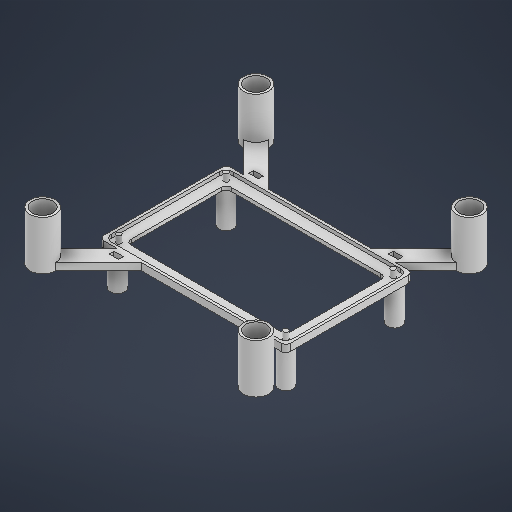
# Autodesk Inventor part: Drone
Saved by Autodesk Inventor 2026 (Build 300175050, 175E)
## iProperties
Created: 2026-01-22
Part Number: Drone
Material: Ogólny
Document SubType Name: Modeling
Designer: DeathLock
Density: 1 g/cm^3
Appearance: Domyślna
Author: DeathLock
Autodesk Inventor part; units mm, degrees
ref_plane "YZ Plane" through (0, 0, 0) normal (1, 0, 0) x (0, 1, 0)
ref_plane "XZ Plane" through (0, 0, 0) normal (0, 1, 0) x (-1, 0, 0)
ref_plane "XY Plane" through (0, 0, 0) normal (0, 0, 1) x (1, 0, 0)
sketch "Szkic1" plane through (0, 0, 0) normal (0, 1, 0) x (-1, 0, 0)
  line L0 (50, 50) -> (-50, 50)
  line L1 (-50, 50) -> (-50, -50)
  line L2 (-50, -50) -> (50, -50)
  line L3 (50, -50) -> (50, 50)
  point P0 (0, 0)
  dimension "d71" = 50
  dimension "d72" = 50
  dimension "d73" = 50
  dimension "d74" = 50
  constraints: 8 end point, 2 parallel, 1 horizontal, 1 perpendicular
  measures "d71" distance from line of L2 point (0, 0)
  measures "d72" distance from line of L3 point (0, 0)
  measures "d73" distance from line of L0 point (0, 0)
  measures "d74" distance from line of L1 point (0, 0)
extrude "Wyciągnięcie proste1" add sketch "Szkic1" along normal blind 3
sketch "Szkic2" plane through (0, 3, 0) normal (0, 1, 0) x (1, 0, 0)
  line L0 (-50, 50) -> (-50, -50) projected
  line L1 (-50, 0) -> (50, 0)
  line L2 (50, -50) -> (50, 50) projected
  line L3 (-38, -25.5) -> (38, -25.5)
  line L4 (38, -25.5) -> (38, 25.5)
  line L5 (38, 25.5) -> (-38, 25.5)
  line L6 (-38, 25.5) -> (-38, -25.5)
  line L7 (-50, -50) -> (50, -50) projected
  line L8 (50, 50) -> (-50, 50) projected
  line L9 (-38, -25.5) -> (-35, -25.5)
  line L10 (-35, -25.5) -> (-35, -22.5)
  line L11 (-35, -22.5) -> (-38, -22.5)
  line L12 (-38, -22.5) -> (-38, -25.5)
  line L13 (-38, 25.5) -> (-35, 25.5)
  line L14 (-35, 25.5) -> (-35, 22.5)
  line L15 (-35, 22.5) -> (-38, 22.5)
  line L16 (-38, 22.5) -> (-38, 25.5)
  line L17 (38, -25.5) -> (35, -25.5)
  line L18 (35, -25.5) -> (35, -22.5)
  line L19 (35, -22.5) -> (38, -22.5)
  line L20 (38, -22.5) -> (38, -25.5)
  line L21 (38, 25.5) -> (35, 25.5)
  line L22 (35, 25.5) -> (35, 22.5)
  line L23 (35, 22.5) -> (38, 22.5)
  line L24 (38, 22.5) -> (38, 25.5)
  circle A0 centre (-35, -22.5) radius 3
  circle A1 centre (-35, 22.5) radius 3
  circle A2 centre (35, 22.5) radius 3
  circle A3 centre (35, -22.5) radius 3
  point P0 (0, 0)
  point P1 (0, -25.5)
  point P2 (0, 25.5)
  point P3 (-38, 0)
  point P4 (38, 0)
  point P5 (-35, -25.5)
  point P6 (38, 22.5)
  dimension "d4" = 76
  dimension "d5" = 51
  dimension "d6" = 24.5
  dimension "d7" = 24.5
  dimension "d8" = 12
  dimension "d9" = 12
  dimension "d10" = 3
  dimension "d11" = 3
  dimension "d12" = 3
  dimension "d13" = 3
  dimension "d14" = 3
  dimension "d15" = 3
  dimension "d16" = 3
  dimension "d17" = 3
  dimension "d75" = 12
  constraints: 42 end point, 10 parallel, 6 midpoint, 5 horizontal, 5 perpendicular, 4 coincident, 12 other
  measures "d4" distance of L5.end L4.end
  measures "d5" distance of L4.end L3.end
  measures "d6" distance from line of L7 point (0, -25.5)
  measures "d7" distance from line of L8 point (0, 25.5)
  measures "d8" distance from line of L0 point (-38, 0)
  measures "d9" distance from line of L2 point (38, 0)
  measures "d10" distance of L11.end L10.end
  measures "d11" distance of L10.end L9.end
  measures "d12" distance of L14.end L15.end
  measures "d13" distance of L13.end L14.end
  measures "d14" distance of L18.end L19.end
  measures "d15" distance of L17.end L18.end
  measures "d16" distance of L23.end L22.end
  measures "d17" distance of L22.end L21.end
  measures "d75" distance between parallel lines of L2 L4
extrude "Wyciągnięcie proste2" cut sketch "Szkic2" against normal blind 1.5 contours L6 A1 L5 A2 L4 L1 | L1 L4 A3 L3 A0 L6 | A1 L14 L15 | L15 L14 A1 | A0 L10 L11 | L11 L10 A0 | A3 L18 L19 | L19 L18 A3 | A2 L22 L23 | L23 L22 A2
sketch "Szkic3" plane through (0, 1.5, 0) normal (0, 1, 0) x (1, 0, 0)
  arc A0 (-38, -22.5) -> (-35, -25.5) centre (-35, -22.5) ccw projected
  arc A1 (38, 22.5) -> (35, 25.5) centre (35, 22.5) ccw projected
  line L0 (-35, -25.5) -> (35, -25.5)
  line L1 (35, -25.5) -> (35, 25.5)
  line L2 (35, 25.5) -> (-35, 25.5)
  line L3 (-35, 25.5) -> (-35, -25.5)
  line L4 (-38, -22.5) -> (-38, 22.5) projected
  line L5 (38, 22.5) -> (-38, 22.5)
  line L6 (-38, 22.5) -> (-38, -22.5)
  line L7 (-38, -22.5) -> (38, -22.5)
  line L8 (38, -22.5) -> (38, 22.5)
  circle A2 centre (-35, -22.5) radius 1
  circle A3 centre (-35, 22.5) radius 1
  circle A4 centre (35, -22.5) radius 1
  circle A5 centre (35, 22.5) radius 1
  point P0 (0, 0)
  dimension "d20" = 2
  dimension "d21" = 2
  dimension "d22" = 2
  dimension "d23" = 2
  constraints: 16 end point, 4 centre point, 4 parallel, 4 point on line, 2 coincident, 2 horizontal, 2 perpendicular
  measures "d20" diameter of A2
  measures "d21" diameter of A3
  measures "d22" diameter of A4
  measures "d23" diameter of A5
extrude "Wyciągnięcie proste3" add sketch "Szkic3" along normal blind 3 contours A2 L3 L7 | L7 L3 A2 | L3 L7 A2 | A3 L3 L5 | L5 L3 A3 | L3 A2 L7 | A4 L7 L1 | L1 L7 A4 | L5 A3 L3 | L3 A3 L5 | L7 A4 L1 | L1 A4 L7 | A5 L1 L5 | L5 L1 A5 | L1 L5 A5 | L1 A5 L5
sketch "Szkic7" plane through (0, 1.5, 0) normal (0, 1, 0) x (1, 0, 0)
  arc A0 (-38, -22.5) -> (-35, -25.5) centre (-35, -22.5) ccw projected
  line L0 (38, 22.5) -> (38, -22.5) projected
  line L1 (-38, -22.5) -> (38, -22.5)
  line L2 (38, -22.5) -> (38, 22.5)
  line L3 (38, 22.5) -> (-38, 22.5)
  line L4 (-38, 22.5) -> (-38, -22.5)
  arc A1 (38, 22.5) -> (35, 25.5) centre (35, 22.5) ccw projected
  line L5 (35, 25.5) -> (-35, 25.5)
  line L6 (-35, 25.5) -> (-35, -25.5)
  line L7 (-35, -25.5) -> (35, -25.5)
  line L8 (35, -25.5) -> (35, 25.5)
  line L9 (-35, -22.5) -> (-32.8787, -20.3787)
  line L10 (-35, -22.5) -> (-32, -22.5) construction
  line L11 (35, 22.5) -> (32.8787, 20.3787)
  line L12 (35, -22.5) -> (32.8787, -20.3787)
  circle A2 centre (-35, 22.5) radius 1 projected
  line L13 (-35, 22.5) -> (-32.8787, 20.3787)
  line L14 (-32.8787, -20.3787) -> (32.8787, -20.3787)
  line L15 (32.8787, -20.3787) -> (32.8787, 20.3787)
  line L16 (32.8787, 20.3787) -> (-32.8787, 20.3787)
  line L17 (-32.8787, 20.3787) -> (-32.8787, -20.3787)
  line L18 (-32.8787, -20.3787) -> (-31.3789, -18.8789)
  circle A3 centre (-31.3789, -18.8789) radius 2.121
  line L19 (-32.8787, 20.3787) -> (-31.3789, 18.8789)
  line L20 (32.8787, 20.3787) -> (31.3789, 18.8789)
  line L21 (32.8787, -20.3787) -> (31.3789, -18.8789)
  circle A4 centre (-31.3789, 18.8789) radius 2.121
  circle A5 centre (31.3789, 18.8789) radius 2.121
  circle A6 centre (31.3789, -18.8789) radius 2.121
  line L22 (31.3789, -20.9999) -> (-31.3789, -20.9999)
  line L23 (-31.3789, -20.9999) -> (-31.3789, 20.9999)
  line L24 (-31.3789, 20.9999) -> (31.3789, 20.9999)
  line L25 (31.3789, 20.9999) -> (31.3789, -20.9999)
  line L26 (-33.4999, 18.8789) -> (33.4999, 18.8789)
  line L27 (33.4999, 18.8789) -> (33.4999, -18.8789)
  line L28 (33.4999, -18.8789) -> (-33.4999, -18.8789)
  line L29 (-33.4999, -18.8789) -> (-33.4999, 18.8789)
  point P0 (0, 0)
  point P1 (-33.4999, -18.8789)
  point P2 (-31.3789, -20.9999)
  point P3 (33.4999, 18.8789)
  point P4 (31.3789, 20.9999)
  dimension "d56" = 3
  dimension "d57" = 45
  dimension "d58" = 3
  dimension "d59" = 3
  dimension "d60" = 3
  dimension "d61" = 2.121
  dimension "d62" = 2.121
  dimension "d63" = 2.121
  dimension "d64" = 2.121
  constraints: 58 end point, 10 parallel, 6 horizontal, 6 point on circle, 5 perpendicular, 4 coincident, 2 centre point, 2 point on line, 1 equal length, 6 other
  measures "d56" distance of L9.start L9.end
  measures "d57" angle of L10 L9
  measures "d58" distance of L11.start L11.end
  measures "d59" distance of L12.start L12.end
  measures "d60" distance of L13.start L13.end
  measures "d61" distance of L9.end L18.end
  measures "d62" distance of L16.end L19.end
  measures "d63" distance of L11.end L20.end
  measures "d64" distance of L14.end L21.end
extrude "Wyciągnięcie proste6" cut sketch "Szkic7" against normal blind 17.5 contours L18 L23 L14 | A3 L28 L17 | L17 L28 L18 | L14 L23 A3 | A6 L25 L14 | L21 L28 L15 | L14 L25 L21 | L15 L28 A6 | L23 L28 A3 L14 | L14 A3 L23 | L28 A3 L17 | L17 A3 L23 L28 | L23 A3 L28 | L29 A4 L17 A3 | A3 L14 A6 L22 | A5 L26 L15 | L20 L25 L16 | L15 L26 L20 | L16 L25 A5 | L25 A6 L14 | L14 A6 L28 L25 | L28 L25 A6 L15 | L15 A6 L28 | L28 A6 L25 | A6 L15 A5 L27 | A4 L23 L16 | L19 L26 L17 | L16 L23 L19 | L17 L26 A4 | A3 L28 A6 L14 | L17 A4 L23 A3 | L23 A4 L26 A5 L25 A6 L28 A3 | L26 L17 A4 | L26 A5 L15 | L15 A5 L25 L26 | L25 L26 A5 L16 | L16 A5 L25 | L25 A5 L26 | A5 L16 A4 L24 | A6 L25 A5 L15 | L23 A4 L16 | L16 A4 L26 L23 | L26 L23 A4 L17 | L26 A4 L23 | A5 L26 A4 L16
sketch "Szkic10" plane through (0, 3, 0) normal (0, 1, 0) x (1, 0, 0)
  line L0 (50, 50) -> (-50, 50) projected
  line L1 (-35, 25.5) -> (35, 25.5) projected
  line L2 (-50, -50) -> (50, -50) projected
  line L3 (35, -25.5) -> (-35, -25.5) projected
  line L4 (50, -50) -> (50, 50) projected
  line L5 (38, 22.5) -> (38, -22.5) projected
  line L6 (-38, -22.5) -> (-38, 22.5) projected
  line L7 (-50, 50) -> (-50, -50) projected
  line L8 (50, 50) -> (44.7, 50)
  line L9 (44.7, 50) -> (44.7, 44.7)
  line L10 (44.7, 44.7) -> (50, 44.7)
  line L11 (50, 44.7) -> (50, 50)
  line L12 (-50, 50) -> (-44.7, 50)
  line L13 (-44.7, 50) -> (-44.7, 44.7)
  line L14 (-44.7, 44.7) -> (-50, 44.7)
  line L15 (-50, 44.7) -> (-50, 50)
  line L16 (-50, -50) -> (-44.7, -50)
  line L17 (-44.7, -50) -> (-44.7, -44.7)
  line L18 (-44.7, -44.7) -> (-50, -44.7)
  line L19 (-50, -44.7) -> (-50, -50)
  line L20 (50, -50) -> (44.7, -50)
  line L21 (44.7, -50) -> (44.7, -44.7)
  line L22 (44.7, -44.7) -> (50, -44.7)
  line L23 (50, -44.7) -> (50, -50)
  circle A0 centre (-44.7, -44.7) radius 5.3
  circle A1 centre (44.7, -44.7) radius 5.3
  circle A2 centre (44.7, 44.7) radius 5.3
  circle A3 centre (-44.7, 44.7) radius 5.3
  circle A4 centre (-44.7, 44.7) radius 4.3
  circle A5 centre (44.7, 44.7) radius 4.3
  circle A6 centre (44.7, -44.7) radius 4.3
  circle A7 centre (-44.7, -44.7) radius 4.3
  point P0 (0, 0)
  dimension "d76" = 24.5
  dimension "d77" = 24.5
  dimension "d78" = 12
  dimension "d79" = 12
  dimension "d80" = 5.3
  dimension "d81" = 5.3
  dimension "d82" = 5.3
  dimension "d83" = 5.3
  dimension "d84" = 5.3
  dimension "d85" = 5.3
  dimension "d86" = 5.3
  dimension "d87" = 5.3
  dimension "d88" = 10.6
  dimension "d89" = 10.6
  dimension "d90" = 10.6
  dimension "d91" = 10.6
  dimension "d92" = 8.6
  dimension "d93" = 8.6
  dimension "d94" = 8.6
  dimension "d95" = 8.6
  constraints: 32 end point, 8 centre point, 8 coincident, 8 parallel, 4 horizontal, 4 perpendicular
  measures "d76" distance between parallel lines of L0 L1
  measures "d77" distance between parallel lines of L2 L3
  measures "d78" distance between parallel lines of L4 L5
  measures "d79" distance between parallel lines of L6 L7
  measures "d80" distance of L10.end L9.end
  measures "d81" distance of L9.end L8.end
  measures "d82" distance of L13.end L14.end
  measures "d83" distance of L12.end L13.end
  measures "d84" distance of L18.end L17.end
  measures "d85" distance of L17.end L16.end
  measures "d86" distance of L21.end L22.end
  measures "d87" distance of L20.end L21.end
  measures "d88" diameter of A0
  measures "d89" diameter of A1
  measures "d90" diameter of A2
  measures "d91" diameter of A3
  measures "d92" diameter of A4
  measures "d93" diameter of A5
  measures "d94" diameter of A6
  measures "d95" diameter of A7
extrude "Wyciągnięcie proste8" add sketch "Szkic10" along normal blind 17.5 contours A2 L10 A5 L9 | L9 A5 L10 A2 | A3 L14 A4 L13 | L13 A4 L14 A3 | A1 L21 A6 L22 | L22 A6 L21 A1 | A0 L17 A7 L18 | L18 A7 L17 A0
sketch "Szkic11" plane through (0, 3, 0) normal (0, 1, 0) x (1, 0, 0)
  arc A0 (-44.7, -50) -> (-50, -44.7) centre (-44.7, -44.7) ccw projected
  arc A1 (-50, -44.7) -> (-44.7, -50) centre (-44.7, -44.7) ccw projected
  line L0 (-40.6047, -41.3357) -> (-44.7, -44.7)
  circle A2 centre (44.7, -44.7) radius 5.3 projected
  line L1 (41.3934, -40.558) -> (44.7, -44.7)
  circle A3 centre (44.7, 44.7) radius 4.3 projected
  line L2 (44.7, 40.4) -> (44.7, 44.7)
  circle A4 centre (-44.7, 44.7) radius 4.3 projected
  line L3 (-48.3948, 42.5003) -> (-44.7, 44.7)
  circle A5 centre (-44.7, 44.7) radius 5.3 projected
  line L4 (-50, 50) -> (-50, 44.7) projected
  arc A6 (-44.7, 50) -> (-50, 44.7) centre (-44.7, 44.7) ccw
  line L5 (50, -50) -> (50, 50) projected
  line L6 (50, 50) -> (44.7, 50) projected
  arc A7 (50, 44.7) -> (44.7, 50) centre (44.7, 44.7) ccw
  arc A8 (44.7, -50) -> (50, -44.7) centre (44.7, -44.7) ccw
  arc A9 (-50, -44.7) -> (-44.7, -50) centre (-44.7, -44.7) ccw
  line L7 (-50, -44.7) -> (-50, -50) projected
  line L8 (-50, -50) -> (-44.7, -50)
  line L9 (-44.7, -50) -> (-44.7, -44.7)
  line L10 (-44.7, -44.7) -> (-50, -44.7)
  line L11 (-50, -44.7) -> (-50, -50)
  line L12 (44.7, -44.7) -> (50, -44.7)
  line L13 (50, -44.7) -> (50, -50)
  line L14 (50, -50) -> (44.7, -50)
  line L15 (44.7, -50) -> (44.7, -44.7)
  line L16 (44.7, 44.7) -> (50, 44.7)
  line L17 (50, 44.7) -> (50, 50)
  line L18 (50, 50) -> (44.7, 50)
  line L19 (44.7, 50) -> (44.7, 44.7)
  line L20 (-50, 50) -> (-44.7, 50)
  line L21 (-44.7, 50) -> (-44.7, 44.7)
  line L22 (-44.7, 44.7) -> (-50, 44.7)
  line L23 (-50, 44.7) -> (-50, 50)
  point P0 (0, 0)
  constraints: 40 end point, 13 point on circle, 8 parallel, 4 centre point, 4 coincident, 4 horizontal, 4 perpendicular, 2 point on line, 1 concentric, 1 vertical, 1 vertical alignment, 3 other
extrude "Wyciągnięcie proste9" cut sketch "Szkic11" against normal blind 17.5 contours L8 L7 A1 | L5 L14 A2 | A7 L6 L5 | L4 L20 A5
sketch "Szkic12" plane through (0, 3, 0) normal (0, 1, 0) x (1, 0, 0)
  circle A0 centre (-44.7, 44.7) radius 4.3 projected
  line L0 (-49, 44.7) -> (-40.4, 44.7)
  arc A1 (44.7, 50) -> (50, 44.7) centre (44.7, 44.7) ccw projected
  line L1 (44.7, 44.7) -> (40.4, 44.7)
  circle A2 centre (44.7, 44.7) radius 4.3 projected
  line L2 (44.7, 44.7) -> (49, 44.7)
  circle A3 centre (44.7, -44.7) radius 4.3 projected
  line L3 (44.7, -44.7) -> (40.4, -44.7)
  line L4 (44.7, -44.7) -> (49, -44.7)
  line L5 (-44.7, -44.7) -> (-40.4, -44.7)
  line L6 (-40.4, -44.7) -> (-44.7, -44.7)
  circle A4 centre (-44.7, -44.7) radius 4.3 projected
  line L7 (-44.7, -44.7) -> (-49, -44.7)
  arc A5 (-50, -44.7) -> (-44.7, -50) centre (-44.7, -44.7) ccw projected
  line L8 (-50, -44.7) -> (-39.4952, -44.7)
  line L9 (-39.4952, -44.7) -> (-39.4952, -43.7)
  line L10 (-39.4952, -43.7) -> (-50, -43.7)
  line L11 (-50, -43.7) -> (-50, -44.7)
  line L12 (-50, -44.7) -> (-39.4952, -44.7)
  line L13 (-39.4952, -44.7) -> (-39.4952, -45.7)
  line L14 (-39.4952, -45.7) -> (-50, -45.7)
  line L15 (-50, -45.7) -> (-50, -44.7)
  arc A6 (50, -44.7) -> (44.7, -50) centre (44.7, -44.7) ccw projected
  line L16 (49, -44.7) -> (39.4952, -44.7)
  line L17 (39.4952, -44.7) -> (39.4952, -43.7)
  line L18 (39.4952, -43.7) -> (49, -43.7)
  line L19 (49, -43.7) -> (49, -44.7)
  line L20 (49, -44.7) -> (39.4952, -44.7)
  line L21 (39.4952, -44.7) -> (39.4952, -45.7)
  line L22 (39.4952, -45.7) -> (49, -45.7)
  line L23 (49, -45.7) -> (49, -44.7)
  line L24 (40.4, 44.7) -> (49.9048, 44.7)
  line L25 (49.9048, 44.7) -> (49.9048, 45.7)
  line L26 (49.9048, 45.7) -> (40.4, 45.7)
  line L27 (40.4, 45.7) -> (40.4, 44.7)
  line L28 (50, -44.7) -> (50, 44.7) projected
  line L29 (40.4, 44.7) -> (50, 44.7)
  line L30 (50, 44.7) -> (50, 43.7)
  line L31 (50, 43.7) -> (40.4, 43.7)
  line L32 (40.4, 43.7) -> (40.4, 44.7)
  line L33 (-49, 44.7) -> (-39.4952, 44.7)
  line L34 (-39.4952, 44.7) -> (-39.4952, 45.7)
  line L35 (-39.4952, 45.7) -> (-49, 45.7)
  line L36 (-49, 45.7) -> (-49, 44.7)
  line L37 (-49, 44.7) -> (-39.4952, 44.7)
  line L38 (-39.4952, 44.7) -> (-39.4952, 43.7)
  line L39 (-39.4952, 43.7) -> (-49, 43.7)
  line L40 (-49, 43.7) -> (-49, 44.7)
  point P0 (0, 0)
  point P1 (-40.5179, -43.7)
  point P2 (-48.8821, -43.7)
  point P3 (-48.8821, -45.7)
  point P4 (-40.5179, -45.7)
  point P5 (48.8821, -43.7)
  point P6 (40.5179, -43.7)
  point P7 (40.5179, -45.7)
  point P8 (48.8821, -45.7)
  point P9 (48.8821, 45.7)
  point P10 (40.5179, 45.7)
  point P11 (40.5179, 43.7)
  point P12 (48.8821, 43.7)
  point P13 (-48.8821, 43.7)
  point P14 (-40.5179, 43.7)
  point P15 (-40.5179, 45.7)
  point P16 (-48.8821, 45.7)
  dimension "d100" = 1
  dimension "d101" = 1
  dimension "d102" = 1
  dimension "d103" = 1
  dimension "d104" = 1
  dimension "d105" = 1
  dimension "d106" = 1
  dimension "d107" = 1
  constraints: 80 end point, 18 equal length, 12 point on circle, 9 horizontal, 9 point on line, 8 perpendicular
  measures "d100" distance of L9.end L8.end
  measures "d101" distance of L12.end L13.end
  measures "d102" distance of L16.end L17.end
  measures "d103" distance of L21.end L20.end
  measures "d104" distance of L25.end L24.end
  measures "d105" distance of L29.end L30.end
  measures "d106" distance of L34.end L33.end
  measures "d107" distance of L37.end L38.end
extrude "Wyciągnięcie proste10" cut sketch "Szkic12" against normal blind 17.5 contours L0 A0 L35 | A0 L39 L0 | L31 A2 L1 L2 | L2 L1 A2 L26 | L4 L3 A3 L18 | A3 L22 L3 L4 | L7 A4 L10 L5 | L5 A4 L14 L7
sketch "Szkic14" plane through (0, 3, 0) normal (0, 1, 0) x (1, 0, 0)
  circle A0 centre (-35, 22.5) radius 1 projected
  line L0 (-35, 22.5) -> (-37.1213, 24.6213)
  arc A1 (-35, 25.5) -> (-38, 22.5) centre (-35, 22.5) ccw projected
  line L1 (-35, 22.5) -> (-32, 22.5) construction
  line L2 (-37.1213, 24.6213) -> (-38.5355, 26.0355)
  line L3 (-37.1213, 24.6213) -> (-35.1213, 24.6213) construction
  circle A2 centre (-37.1213, 24.6213) radius 2
  arc A3 (38, 22.5) -> (35, 25.5) centre (35, 22.5) ccw projected
  circle A4 centre (37.1213, 24.6213) radius 2
  arc A5 (35, -25.5) -> (38, -22.5) centre (35, -22.5) ccw projected
  circle A6 centre (37.1213, -24.6213) radius 2
  arc A7 (-38, -22.5) -> (-35, -25.5) centre (-35, -22.5) ccw projected
  circle A8 centre (-37.1213, -24.6213) radius 2
  line L4 (-39.1213, -24.6213) -> (-39.1213, 24.6213)
  line L5 (-37.1213, 26.6213) -> (37.1213, 26.6213)
  line L6 (39.1213, 24.6213) -> (39.1213, -24.6213)
  line L7 (37.1213, -26.6213) -> (-37.1213, -26.6213)
  line L8 (-50, 44.7) -> (-50, -44.7) projected
  line L9 (50, -44.7) -> (50, 44.7) projected
  line L10 (-50, 44.7) -> (50, 44.7)
  line L11 (50, 44.7) -> (50, -44.7)
  line L12 (50, -44.7) -> (-50, -44.7)
  line L13 (-50, -44.7) -> (-50, 44.7)
  circle A9 centre (44.7, -44.7) radius 5.3 projected
  circle A10 centre (-44.7, 44.7) radius 5.3 projected
  line L14 (44.7, -50) -> (-44.7, -50)
  line L15 (-44.7, -50) -> (-44.7, 50)
  line L16 (-44.7, 50) -> (44.7, 50)
  line L17 (44.7, 50) -> (44.7, -50)
  circle A11 centre (-44.7, -44.7) radius 5.3
  circle A12 centre (44.7, -44.7) radius 5.3
  circle A13 centre (44.7, 44.7) radius 5.3
  circle A14 centre (-44.7, 44.7) radius 5.3
  line L18 (-32, -26.6213) -> (-21.3769, -26.6213)
  line L19 (-44.7, -39.4) -> (-34, -39.4)
  arc A15 (-48.8821, -43.7) -> (-48.8821, -45.7) centre (-44.7, -44.7) ccw projected
  line L20 (-48.8821, -43.7) -> (-43.7, -48.8821)
  arc A16 (-48.8821, -45.7) -> (-40.5179, -45.7) centre (-44.7, -44.7) ccw projected
  circle A17 centre (-44.7, 44.7) radius 4.3 projected
  line L21 (-48.8821, 43.7) -> (-43.7, 48.8821)
  circle A18 centre (44.7, 44.7) radius 4.3 projected
  line L22 (43.7, 48.8821) -> (48.8821, 43.7)
  circle A19 centre (44.7, -44.7) radius 4.3 projected
  line L23 (43.7, -48.8821) -> (48.8821, -43.7)
  line L24 (-44.7, 39.4) -> (39.4, -44.7)
  line L25 (44.7, -39.4) -> (-39.4, 44.7)
  line L26 (39.4, 44.7) -> (-44.7, -39.4)
  line L27 (-39.4, -44.7) -> (44.7, 39.4)
  point P0 (0, 0)
  point P1 (31.9213, -26.6213)
  point P2 (31.9213, 26.6213)
  point P3 (21.3213, 26.6213)
  point P4 (-39.4, 44.7)
  point P5 (-21.3213, 26.6213)
  point P6 (21.3213, -26.6213)
  point P7 (-21.3213, -26.6213)
  point P8 (-31.9213, -26.6213)
  point P9 (-31.9213, 26.6213)
  point P10 (-44.7, 39.4)
  point P11 (-50, -44.7)
  dimension "d118" = 135
  dimension "d119" = 2
  dimension "d120" = 135
  dimension "d121" = 4
  dimension "d122" = 4
  dimension "d123" = 4
  constraints: 52 end point, 30 point on circle, 13 point on line, 8 centre point, 6 parallel, 6 tangent, 5 perpendicular, 4 horizontal, 3 coincident, 2 concentric, 2 equal length, 1 collinear
  measures "d118" angle of L1 L0
  measures "d119" distance of L0.end L2.end
  measures "d120" angle of L3 L2
  measures "d121" diameter of A4
  measures "d122" diameter of A6
  measures "d123" diameter of A8
extrude "Wyciągnięcie proste11" cut sketch "Szkic14" against normal blind 17.5 contours A2 L4 A8 L7 L26 L15 L24 L5 | L25 L10 L26 L5 | L15 A11 L8 A10 | A10 L16 A13 L10 | L27 L17 L25 L7 A6 L6 A4 L5 | L27 L7 L24 L12 | L12 A9 L14 A11 | A13 L9 A9 L17
sketch "Szkic15" plane through (0, 3, 0) normal (0, 1, 0) x (1, 0, 0)
  line L0 (-31.9213, -26.6213) -> (-37.1213, -26.6213) projected
  line L1 (-21.3213, -26.6213) -> (-39.4, -44.7) projected
  line L2 (-31.9213, -26.6213) -> (-39.4, -26.6213)
  line L3 (-39.4, -26.6213) -> (-39.4, -44.7)
  line L4 (-39.4, -44.7) -> (-31.9213, -44.7)
  line L5 (-31.9213, -44.7) -> (-31.9213, -26.6213)
  line L6 (-21.3213, -26.6213) -> (-44.7, -26.6213)
  line L7 (-44.7, -26.6213) -> (-44.7, -39.4)
  line L8 (-44.7, -39.4) -> (-21.3213, -39.4)
  line L9 (-21.3213, -39.4) -> (-21.3213, -26.6213)
  line L10 (-31.9213, -26.6213) -> (-26.6213, -26.6213)
  line L11 (-26.6213, -26.6213) -> (-39.4, -39.4)
  line L12 (-26.6213, -26.6213) -> (-26.6213, -31.9213)
  line L13 (-31.9213, -26.6213) -> (-26.6213, -31.9213)
  line L14 (-29.2713, -29.2713) -> (-34.5713, -29.2713)
  line L15 (-31.9213, -26.6213) -> (-44.7, -39.4) projected
  line L16 (-29.2713, -29.2713) -> (-23.9713, -29.2713)
  line L17 (-31.2713, -28.2713) -> (-27.2713, -28.2713)
  line L18 (-27.2713, -28.2713) -> (-27.2713, -30.2713)
  line L19 (-27.2713, -30.2713) -> (-31.2713, -30.2713)
  line L20 (-31.2713, -30.2713) -> (-31.2713, -28.2713)
  arc A0 (44.7, -39.4) -> (39.4, -44.7) centre (44.7, -44.7) ccw projected
  line L21 (31.9213, -26.6213) -> (39.4, -26.6213)
  line L22 (39.4, -26.6213) -> (39.4, -44.7)
  line L23 (39.4, -44.7) -> (31.9213, -44.7)
  line L24 (31.9213, -44.7) -> (31.9213, -26.6213)
  line L25 (39.4, -44.7) -> (21.3213, -26.6213) projected
  line L26 (44.7, -39.4) -> (21.3213, -39.4)
  line L27 (21.3213, -39.4) -> (21.3213, -26.6213)
  line L28 (21.3213, -26.6213) -> (44.7, -26.6213)
  line L29 (44.7, -26.6213) -> (44.7, -39.4)
  line L30 (-34.5713, -29.2713) -> (34.5713, -29.2713)
  line L31 (44.7, -39.4) -> (31.9213, -26.6213) projected
  line L32 (21.3213, -26.6213) -> (26.6213, -26.6213)
  line L33 (26.6213, -26.6213) -> (39.4, -39.4)
  line L34 (31.2713, -28.2713) -> (27.2713, -28.2713)
  line L35 (27.2713, -28.2713) -> (27.2713, -30.2713)
  line L36 (27.2713, -30.2713) -> (31.2713, -30.2713)
  line L37 (31.2713, -30.2713) -> (31.2713, -28.2713)
  line L38 (29.2713, -29.2713) -> (29.2713, -28.2713)
  line L39 (31.9213, -26.6213) -> (31.9213, 37.2213)
  line L40 (39.4, 44.7) -> (21.3213, 26.6213) projected
  line L41 (31.2713, -28.2713) -> (31.2713, 36.5713)
  line L42 (31.2713, -28.2713) -> (96.114, -28.2713) construction
  line L43 (27.2713, -28.2713) -> (27.2713, 32.5713)
  line L44 (27.2713, -28.2713) -> (88.114, -28.2713) construction
  line L45 (21.3213, 26.6213) -> (31.9213, 26.6213)
  line L46 (27.2713, 26.6213) -> (27.2713, 28.2713)
  line L47 (27.2713, 28.2713) -> (31.2713, 28.2713)
  line L48 (31.2713, 28.2713) -> (31.2713, 30.2713)
  line L49 (31.2713, 30.2713) -> (27.2713, 30.2713)
  line L50 (27.2713, 30.2713) -> (27.2713, 28.2713)
  line L51 (-31.2713, -28.2713) -> (-31.2713, 36.5713)
  line L52 (-31.2713, -28.2713) -> (33.5713, -28.2713) construction
  line L53 (-27.2713, -28.2713) -> (-27.2713, 32.5713)
  line L54 (-39.4, 44.7) -> (-21.3213, 26.6213) projected
  line L55 (-27.2713, -28.2713) -> (33.5713, -28.2713) construction
  line L56 (27.2713, 30.2713) -> (-31.2713, 30.2713)
  line L57 (27.2713, 30.2713) -> (85.814, 30.2713) construction
  line L58 (27.2713, 28.2713) -> (-31.2713, 28.2713)
  point P0 (0, 0)
  point P1 (-29.2713, -30.2713)
  point P2 (-27.2713, 28.2713)
  point P3 (-27.2713, 30.2713)
  dimension "d126" = 5.3
  dimension "d127" = 2
  dimension "d128" = 1
  dimension "d129" = 2
  dimension "d130" = 1
  dimension "d131" = 5.3
  dimension "d132" = 1
  dimension "d133" = 1
  dimension "d134" = 2
  dimension "d135" = 2
  dimension "d136" = 90
  dimension "d137" = 90
  dimension "d138" = 1.65
  dimension "d139" = 4
  dimension "d140" = 2
  dimension "d141" = 90
  dimension "d142" = 90
  dimension "d143" = 180
  constraints: 104 end point, 22 point on line, 14 parallel, 13 horizontal, 11 perpendicular, 5 equal length, 3 midpoint, 2 vertical
  measures "d126" distance of L0.start L10.end
  measures "d127" distance from line of L20 L14.start
  measures "d128" distance from line of L17 L14.start
  measures "d129" distance from line of L18 L14.start
  measures "d130" distance of point (-29.271, -30.271) L14.start
  measures "d131" distance of L25.end L32.end
  measures "d132" distance between parallel lines of L34 L30
  measures "d133" distance between parallel lines of L30 L36
  measures "d134" distance from line of L35 L38.start
  measures "d135" distance from line of L37 L38.start
  measures "d136" angle of L42 L41
  measures "d137" angle of L44 L43
  measures "d138" distance of L46.start L46.end
  measures "d139" distance of L49.end L48.end
  measures "d140" distance of L48.end L47.end
  measures "d141" angle of L52 L51
  measures "d142" angle of L55 L53
  measures "d143" angle of L56 L57
extrude "Wyciągnięcie proste12" cut sketch "Szkic15" against normal blind 17.5 contours L20 L17 L13 L14 | L14 L11 L19 L20 | L51 L56 L53 L58 | L17 L11 L13 | L11 L13 L19 | L16 L18 L19 L13 | L11 L17 L18 L16 | L43 L49 L41 L47 | L35 L34 L33 L30 | L30 L33 L36 L35 | L38 L34 L37 L30 | L30 L37 L36 L33 | L33 L34 L38
sketch "Szkic17" plane through (0, 0, 0) normal (0, -1, 0) x (1, 0, 0)
  arc A0 (-31.3789, 20.9999) -> (-33.4999, 18.8789) centre (-31.3789, 18.8789) ccw projected
  line L0 (-33.4999, 18.8789) -> (-31.3789, 18.8789)
  line L1 (-31.3789, 18.8789) -> (-31.3789, 20.9999)
  line L2 (-37.1213, 26.6213) -> (-31.9213, 26.6213) projected
  arc A1 (-37.1213, 26.6213) -> (-39.1213, 24.6213) centre (-37.1213, 24.6213) ccw projected
  line L3 (-37.1213, 26.6213) -> (-39.1213, 26.6213)
  line L4 (-39.1213, 26.6213) -> (-39.1213, 24.6213)
  arc A2 (33.4999, 18.8789) -> (31.3789, 20.9999) centre (31.3789, 18.8789) ccw projected
  arc A3 (39.1213, 24.6213) -> (37.1213, 26.6213) centre (37.1213, 24.6213) ccw projected
  line L5 (39.1213, 20.9999) -> (39.1213, 24.6213)
  line L6 (31.3789, 24.6213) -> (31.3789, 20.9999)
  line L7 (33.4999, -18.8789) -> (33.4999, 18.8789) projected
  line L8 (37.1213, 26.6213) -> (33.4999, 26.6213)
  line L9 (33.4999, 18.8789) -> (37.1213, 18.8789)
  line L10 (39.1213, -21.0056) -> (39.1213, -24.7715)
  line L11 (31.3789, -24.7715) -> (31.3789, -21.0056)
  arc A4 (31.3789, -20.9999) -> (33.4999, -18.8789) centre (31.3789, -18.8789) ccw projected
  arc A5 (37.1213, -26.6213) -> (39.1213, -24.6213) centre (37.1213, -24.6213) ccw projected
  line L12 (33.4999, -18.8789) -> (37.1213, -18.8789)
  line L13 (37.1213, -26.6213) -> (33.4999, -26.6213)
  arc A6 (-33.4999, -18.8789) -> (-31.3789, -20.9999) centre (-31.3789, -18.8789) ccw projected
  line L14 (-39.1213, -20.9999) -> (-39.1213, -24.7715)
  line L15 (-31.3789, -24.7715) -> (-31.3789, -20.9999)
  line L16 (-33.4999, -18.8789) -> (-37.1213, -18.8789)
  line L17 (-37.1213, -26.6213) -> (-33.4999, -26.6213)
  line L18 (-37.1213, 26.6213) -> (-33.4999, 26.6213)
  line L19 (-33.4999, 18.8789) -> (-37.1213, 18.8789)
  line L20 (-39.1213, 20.9999) -> (-39.1213, 24.6213)
  line L21 (-31.3789, 24.6213) -> (-31.3789, 20.9999)
  circle A7 centre (-35.2501, 22.8106) radius 3
  circle A8 centre (35.3106, 22.8106) radius 3
  circle A9 centre (35.3106, -22.7501) radius 3
  circle A10 centre (-35.3106, -22.7501) radius 3
  point P0 (0, 0)
  dimension "d146" = 6
  dimension "d147" = 6
  dimension "d148" = 6
  dimension "d149" = 6
  constraints: 40 end point, 8 parallel, 5 horizontal, 4 centre point, 4 point on line, 1 perpendicular
  measures "d146" diameter of A7
  measures "d147" diameter of A8
  measures "d148" diameter of A9
  measures "d149" diameter of A10
extrude "Wyciągnięcie proste13" add sketch "Szkic17" along normal blind 15 contours A7 | A8 | A9 | A10
sketch "Szkic18" plane through (35.3106, -15, 22.8106) normal (0, -1, 0) x (1, 0, 0)
  circle A0 centre (0, 0) radius 2
  circle A1 centre (-70.5607, 0) radius 3 projected
  circle A2 centre (-70.5607, 0) radius 2
  circle A3 centre (0, -45.5607) radius 3 projected
  circle A4 centre (0, -45.5607) radius 2
  circle A5 centre (-70.5607, -45.5607) radius 2
  point P0 (-35.3106, -22.8106)
  dimension "d152" = 4
  dimension "d153" = 4
  dimension "d154" = 4
  dimension "d155" = 4
  constraints: 4 centre point, 2 coincident
  measures "d152" diameter of A0
  measures "d153" diameter of A2
  measures "d154" diameter of A4
  measures "d155" diameter of A5
extrude "Wyciągnięcie proste14" cut sketch "Szkic18" against normal blind 15 contours A0 | A2 | A4 | A5
